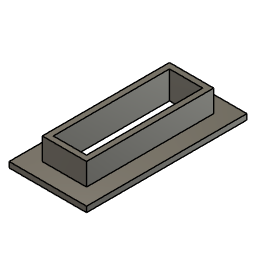
interrupteur v4 (Autodesk Fusion 360 design; units mm, degrees)
Autodesk Fusion 360 part; units mm, degrees
sketch "Esquisse1" plane through (0, 0, 0) normal (0, 1, 0) x (1, 0, 0)
  line L0 (0, 0) -> (6, 0)
  line L1 (6, 0) -> (6, -21)
  line L2 (6, -21) -> (0, -21)
  line L3 (0, -21) -> (0, 0)
  line L4 (-1, 1) -> (7, 1)
  line L5 (7, 1) -> (7, -22)
  line L6 (7, -22) -> (-1, -22)
  line L7 (-1, -22) -> (-1, 1)
  line L8 (-4, 4) -> (10, 4)
  line L9 (10, 4) -> (10, -25)
  line L10 (10, -25) -> (-4, -25)
  line L11 (-4, -25) -> (-4, 4)
  dimension "d1" = 6
  dimension "d2" = 21
  dimension "d3" = 1
  dimension "d4" = 1
  dimension "d5" = 1
  dimension "d6" = 1
  dimension "d7" = 3
  dimension "d8" = 3
  dimension "d9" = 3
  dimension "d10" = 3
  constraint horizontal L0
  constraint vertical L1
  constraint horizontal L2
  constraint vertical L3
  constraint coincident L0.start L3.end
  constraint horizontal L4
  constraint vertical L5
  constraint horizontal L6
  constraint vertical L7
  constraint horizontal L8
  constraint vertical L9
  constraint horizontal L10
  constraint vertical L11
  measures "d1" distance of L0.start L0.end
  measures "d2" distance of L0.start L2.end
  measures "d3" distance of L0 L4
  measures "d4" distance of L2 L6
  measures "d5" distance of L1 L5
  measures "d6" distance of L3 L7
  measures "d7" distance of L4 L8
  measures "d8" distance of L6 L10
  measures "d9" distance of L5 L9
  measures "d10" distance of L7 L11
extrude "Extrusion1" add sketch "Esquisse1" along normal blind 5 contours L4 L5 L6 L7
extrude "Extrusion2" add sketch "Esquisse1" along normal blind 1 contours L8 L9 L10 L11
